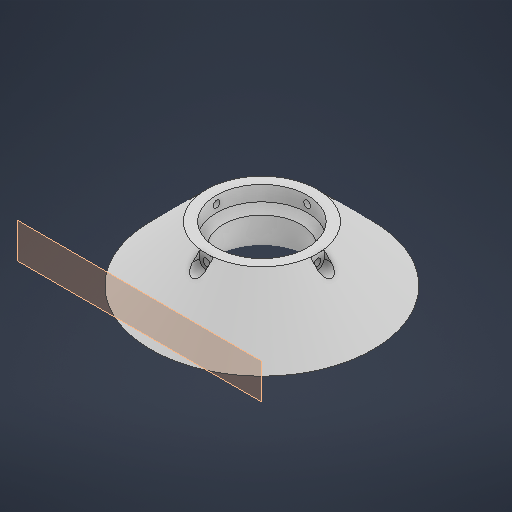
# Autodesk Inventor part: Статор без зубьев
Saved by Autodesk Inventor 2026 (Build 300175000, 175)
## iProperties
Created: 2025-08-22
Part Number: Статор без зубьев
Material: Типовые
Document SubType Name: Modeling
Designer: kvm13
Density: 1 g/cm^3
Appearance: По умолчанию
Author: kvm13
Autodesk Inventor part; units mm, degrees
ref_plane "YZ Plane" through (0, 0, 0) normal (1, 0, 0) x (0, 1, 0)
ref_plane "XZ Plane" through (0, 0, 0) normal (0, 1, 0) x (-1, 0, 0)
sketch "Эскиз1" plane through (0, 0, 0) normal (1, 0, 0) x (0, 1, 0)
  line L0 (0, 0) -> (0, 11.5)
  line L1 (0, 11.5) -> (0, 13.5)
  line L2 (0, 13.5) -> (2, 13.5)
  line L3 (2, 13.5) -> (0, 11.5)
  line L4 (2, 13.5) -> (6.5, 13.5)
  line L5 (6.5, 13.5) -> (6.5, 16.5)
  line L6 (6.5, 16.5) -> (2, 16.5)
  line L7 (0, 13.5) -> (0, 16.5)
  line L8 (0, 16.5) -> (2, 16.5)
  line L9 (6.5, 16.5) -> (-10, 33)
  line L10 (6.5, 16.5) -> (32.9156, 16.5) construction
  line L11 (0, 33) -> (-10, 33)
  line L12 (-10, 33) -> (-10, 16.5)
  line L13 (-10, 16.5) -> (-9.9702, 14.7974) construction
  line L14 (-9.9702, 14.7974) -> (-9.629, 12.8623) construction
  line L15 (-9.629, 12.8623) -> (-8.0037, 11.5) construction
  line L16 (-8.0037, 11.5) -> (0, 11.5) construction
  spline S0 degree 4 poles (-10, 16.5) (-9.9702, 14.7974) (-9.629, 12.8623) (-8.0037, 11.5) (0, 11.5) knots 1 1 1 1 1 2 2 2 2 2
  line L17 (0, 0) -> (14.3588, 0)
  dimension "d1" = 2
  dimension "d2" = 2
  dimension "d3" = 13.5
  dimension "d4" = 3
  dimension "d5" = 4.5
  dimension "d6" = 16.5
  dimension "d7" = 135
  constraints: 28 end point, 5 perpendicular, 4 point on line, 3 horizontal, 2 vertical, 3 other
  measures "d1" distance of L0.end L1.end
  measures "d2" distance of L1.end L2.end
  measures "d3" distance of L0.start L1.end
  measures "d4" distance of L2.end L6.end
  measures "d5" distance of L2.end L4.end
  measures "d6" distance of L7.end L11.start
  measures "d7" angle of L10 L9
revolve "Вращение1" add sketch "Эскиз1" angle 360 about axis through (0, 0, 0) along (0, 1, 0)
sketch "Эскиз2" plane through (0, 0, 0) normal (0, 0, 1) x (1, 0, 0)
  line L0 (13.5, 6.5) -> (-13.5, 6.5) projected
  line L1 (13.5, 2) -> (-13.5, 2) projected
  line L2 (0, 2) -> (0, 6.5)
  circle A0 centre (0, 4.25) radius 1
  point P0 (0, 0)
  dimension "d9" = 2
  constraints: 3 midpoint, 2 end point, 1 centre point
  measures "d9" diameter of A0
extrude "Выдавливание1" cut sketch "Эскиз2" along normal blind 30
ref_plane "РабПлоскость1" through (0, 0, 36.5125) normal (0, 0, 1) x (1, 0, 0)
sketch "Эскиз3" plane through (0, 0, 36.5125) normal (0, 0, 1) x (1, 0, 0)
  line L0 (16.5, 6.5) -> (-16.5, 6.5) projected
  arc A0 (-2, 4.25) -> (2, 4.25) centre (0, 4.25) ccw
  line L1 (-2, 4.25) -> (-2, 6.5)
  line L2 (2, 4.25) -> (2, 6.5)
  point P0 (0, 0)
  point P1 (0.9986, 4.3033)
  dimension "d14" = 4
  constraints: 4 end point, 2 perpendicular, 2 point on circle, 2 point on line, 2 tangent, 1 centre point, 1 other
  measures "d14" diameter of A0
extrude "Выдавливание2" cut sketch "Эскиз3" against normal blind 20.013
pattern_circular "Круговой массив1" count 4 over 360 about axis through (0, 4.25, 0) along (0, 1, 0) of "Выдавливание2", "Выдавливание1"
